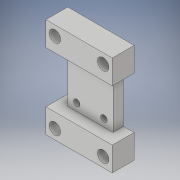
# Autodesk Inventor part: xy 조인트
Saved by Autodesk Inventor 2018 (Build 220112000, 112)
## iProperties
Created: 2019-01-21
Part Number: xy 조인트
Material: Generic
Document SubType Name: Modeling
Designer: User
Density: 1 g/cm^3
Appearance: Default
Author: User
Autodesk Inventor part; units mm, degrees
ref_plane "YZ Plane" through (0, 0, 0) normal (1, 0, 0) x (0, 1, 0)
ref_plane "XZ Plane" through (0, 0, 0) normal (0, 1, 0) x (-1, 0, 0)
ref_plane "XY Plane" through (0, 0, 0) normal (0, 0, 1) x (1, 0, 0)
sketch "스케치1" plane through (0, 0, 0) normal (1, 0, 0) x (0, 1, 0)
  line L0 (-15.9064, 9.3186) -> (-7.9064, 9.3186)
  line L1 (-7.9064, 9.3186) -> (-3.9064, 13.3186)
  line L2 (-3.9064, 13.3186) -> (4.0936, 13.3186)
  line L3 (4.0936, 13.3186) -> (8.0936, 9.3186)
  line L4 (8.0936, 9.3186) -> (16.0936, 9.3186)
  line L5 (-15.9064, -1.1814) -> (-16.9064, -2.1814)
  line L6 (-16.9064, -2.1814) -> (-16.9064, -7.1814)
  line L7 (-16.9064, -7.1814) -> (-15.9064, -8.1814)
  line L8 (16.0936, 9.3186) -> (16.0936, -1.1814)
  line L9 (16.0936, -1.1814) -> (17.0936, -2.1814)
  line L10 (17.0936, -2.1814) -> (17.0936, -7.1814)
  line L11 (17.0936, -7.1814) -> (16.0936, -8.1814)
  line L12 (16.0936, -8.1814) -> (-15.9064, -8.1814) construction
  line L13 (-15.9064, -8.6814) -> (16.0936, -8.6814) construction
  line L14 (-15.9064, -8.1814) -> (-15.4064, -8.6814)
  line L15 (-15.4064, -8.6814) -> (-4.4064, -8.6814)
  line L16 (-4.4064, -8.6814) -> (-3.9064, -8.1814)
  line L17 (-3.9064, -8.1814) -> (4.0936, -8.1814)
  line L18 (4.0936, -8.1814) -> (4.5936, -8.6814)
  line L19 (16.0936, -8.1814) -> (15.5936, -8.6814)
  line L20 (15.5936, -8.6814) -> (4.5936, -8.6814)
  line L21 (-11.9064, 9.3186) -> (-11.9064, 8.0705)
  line L22 (16.0936, 8.8186) -> (33.0936, 8.8186)
  line L23 (33.0936, 8.8186) -> (33.0936, -1.1814)
  line L24 (33.0936, -1.1814) -> (16.0936, -1.1814)
  line L25 (17.0936, -1.1814) -> (17.0936, -8.6814)
  line L26 (17.0936, -8.6814) -> (33.0936, -8.6814)
  line L27 (33.0936, -8.6814) -> (33.0936, -1.1814)
  line L28 (-15.9064, 8.8186) -> (-32.9064, 8.8186)
  line L29 (-32.9064, 8.8186) -> (-32.9064, -1.1814)
  line L30 (-32.9064, -1.1814) -> (-15.9064, -1.1814)
  line L31 (-15.9064, -1.1814) -> (-15.9064, 9.3186)
  line L32 (-16.9064, -1.1814) -> (-16.9064, -8.6814)
  line L33 (-16.9064, -8.6814) -> (-32.9064, -8.6814)
  line L34 (-32.9064, -8.6814) -> (-32.9064, -1.1814)
  line L35 (17.0936, -8.6814) -> (15.5936, -8.6814)
  line L36 (-16.9064, -8.6814) -> (-15.4064, -8.6814)
  line L37 (-4.4064, -8.6814) -> (4.5936, -8.6814)
  line L38 (-32.9064, -8.6814) -> (-32.9064, -15.6814)
  line L39 (-32.9064, -15.6814) -> (33.0936, -15.6814)
  line L40 (33.0936, -15.6814) -> (33.0936, -8.6814)
  line L41 (17.0936, -8.6814) -> (17.0936, -15.6814)
  line L42 (-16.9064, -8.6814) -> (-16.9064, -15.6814)
  point P0 (0, 0)
  dimension "d0" = 8
  dimension "d1" = 135
  dimension "d2" = 135
  dimension "d3" = 4
  dimension "d4" = 8
  dimension "d5" = 8
  dimension "d6" = 135
  dimension "d7" = 135
  dimension "d8" = 10.5
  dimension "d10" = 135
  dimension "d11" = 1
  dimension "d12" = 1
  dimension "d13" = 135
  dimension "d14" = 135
  dimension "d15" = 135
  dimension "d16" = 1
  dimension "d17" = 10.5
  dimension "d18" = 5
  dimension "d19" = 5
  dimension "d20" = 0.5
  dimension "d21" = 11
  dimension "d22" = 8
  dimension "d23" = 135
  dimension "d24" = 135
  dimension "d25" = 135
  dimension "d26" = 135
  dimension "d27" = 135
  dimension "d28" = 11
  dimension "d29" = 10
  dimension "d30" = 17
  dimension "d32" = 17
  constraints: 86 end point, 14 point on line, 11 perpendicular, 3 collinear, 2 vertical, 1 midpoint
  measures "d0" distance of L0.start L0.end
  measures "d1" angle of L0 L1
  measures "d2" angle of L2 L1
  measures "d3" distance from line of L0.end L2
  measures "d4" distance of L1.end L2.end
  measures "d5" distance of L3.end L4.end
  measures "d6" angle of L2 L3
  measures "d7" angle of L3 L4
  measures "d8" distance of L0.start L5.start
  measures "d10" angle of L6 L5
  measures "d11" distance from line of L5.start L6
  measures "d12" distance from line of L9.start L10
  measures "d13" angle of L8 L9
  measures "d14" angle of L9 L10
  measures "d15" angle of L10 L11
  measures "d16" distance from line of L10 L19.start
  measures "d17" distance of L4.end L9.start
  measures "d18" distance of L5.end L6.end
  measures "d19" distance of L10.start L11.start
  measures "d20" distance between parallel lines of L12 L13
  measures "d21" distance of L15.start L16.start
  measures "d22" distance of L17.start L18.start
  measures "d23" angle of L12 L18
  measures "d24" angle of L13 L18
  measures "d25" angle of L13 L19
  measures "d26" angle of L15 L16
  measures "d27" angle of L14 L15
  measures "d28" distance of L20.start L18.end
  measures "d29" distance of L9.start L22.start
  measures "d30" distance of L22.start L22.end
  measures "d32" distance of L28.start L28.end
extrude "돌출2" add sketch "스케치1" along normal blind 30 contours L36 L15 L37 L20 L35 L41 L39 L42
sketch "스케치3" plane through (0, -16.9064, -15.6814) normal (0, 0, -1) x (-1, 0, 0)
  line L0 (0, 34) -> (-30, 34) projected
  line L1 (-30, 0) -> (-30, 34) projected
  line L2 (-30, 34) -> (-30, 29)
  line L3 (-30, 29) -> (-24, 29)
  circle A0 centre (-24, 29) radius 2.15
  line L4 (-30, 0) -> (-30, 5)
  line L5 (-30, 5) -> (-24, 5)
  circle A1 centre (-24, 5) radius 2.15
  line L6 (0, 34) -> (0, 29)
  line L7 (0, 29) -> (-6, 29)
  circle A2 centre (-6, 29) radius 2.15
  line L8 (0, 0) -> (0, 5)
  line L9 (0, 0) -> (0, 34) projected
  line L10 (0, 5) -> (-6, 5)
  circle A3 centre (-6, 5) radius 2.15
  line L11 (0, 34) -> (0, 43.5)
  line L12 (-30, 43.5) -> (-30, 34)
  line L13 (-15, 34) -> (-15, 43.5)
  line L14 (-15, 43.5) -> (1, 43.5)
  line L15 (-15, 43.5) -> (-31, 43.5)
  circle A4 centre (1, 43.5) radius 3.8
  circle A5 centre (-31, 43.5) radius 3.8
  line L16 (0, 0) -> (0, -9.5)
  line L17 (-15, -9.5) -> (-15, 0)
  line L18 (-30, -9.5) -> (-30, 0)
  line L19 (-15, -9.5) -> (-31, -9.5)
  line L20 (-15, -9.5) -> (1, -9.5)
  circle A6 centre (-31, -9.5) radius 3.8
  circle A7 centre (1, -9.5) radius 3.8
  point P0 (0, 16.9064)
  dimension "d38" = 5
  dimension "d39" = 6
  dimension "d40" = 4.3
  dimension "d41" = 5
  dimension "d42" = 6
  dimension "d43" = 4.3
  dimension "d44" = 5
  dimension "d45" = 6
  dimension "d46" = 4.3
  dimension "d47" = 5
  dimension "d48" = 6
  dimension "d49" = 4.3
  dimension "d54" = 9.5
  dimension "d55" = 16
  dimension "d56" = 16
  dimension "d57" = 7.6
  dimension "d58" = 7.6
  dimension "d61" = 9.5
  dimension "d62" = 15
  dimension "d67" = 16
  dimension "d68" = 16
  dimension "d69" = 7.6
  dimension "d70" = 7.6
  constraints: 36 end point, 8 centre point, 8 coincident, 4 horizontal, 3 perpendicular, 3 point on line, 3 vertical, 1 midpoint
  measures "d38" distance of L0.end L2.end
  measures "d39" distance of L2.end L3.end
  measures "d40" diameter of A0
  measures "d41" distance of L1.start L4.end
  measures "d42" distance of L4.end L5.end
  measures "d43" diameter of A1
  measures "d44" distance of L0.start L6.end
  measures "d45" distance of L6.end L7.end
  measures "d46" diameter of A2
  measures "d47" distance of L8.start L8.end
  measures "d48" distance of L8.end L10.end
  measures "d49" diameter of A3
  measures "d54" distance of L0.start L11.end
  measures "d55" distance of L13.end L14.end
  measures "d56" distance of L13.end L15.end
  measures "d57" diameter of A4
  measures "d58" diameter of A5
  measures "d61" distance of L8.start L16.end
  measures "d62" distance of L16.end L17.start
  measures "d67" distance of L17.start L19.end
  measures "d68" distance of L17.start L20.end
  measures "d69" diameter of A6
  measures "d70" diameter of A7
extrude "돌출3" add sketch "스케치1" along normal blind 37 and the other way blind 7 contours L30 L32 L6 L33 L34 | L33 L42 L39 L38 | L41 L26 L40 L39 | L25 L10 L24 L27 L26
extrude "돌출4" cut sketch "스케치3" against normal blind 10 contours A0 | A1 | A3 | A2
extrude "돌출6" cut sketch "스케치3" against normal blind 20 contours A4 L14 L11 | L11 L14 A4 | A5 L15 L12 | L12 L15 A5 | A7 L20 L16 | L16 L20 A7 | A6 L19 L18 | L18 L19 A6
equation "\"d14\" = d13"
equation "\"d15\" = d13"
equation "\"d17\" = d8"
